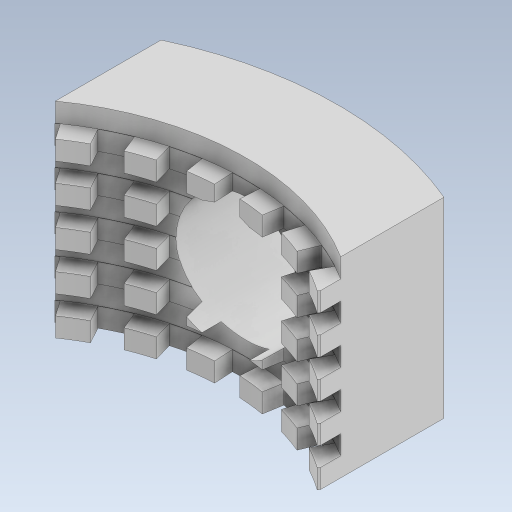
# Autodesk Inventor part: Plunger Cap
Saved by Autodesk Inventor 2023 (Build 270158000, 158)
## iProperties
Created: 2022-09-14
Part Number: Plunger Cap
Material: Generic
Document SubType Name: Modeling
Designer: Dave
Density: 1 g/cm^3
Appearance: Default
Author: Dave
Autodesk Inventor part; units mm, degrees
ref_plane "YZ Plane" through (0, 0, 0) normal (1, 0, 0) x (0, 1, 0)
ref_plane "XZ Plane" through (0, 0, 0) normal (0, 1, 0) x (-1, 0, 0)
ref_plane "XY Plane" through (0, 0, 0) normal (0, 0, 1) x (1, 0, 0)
sketch "Sketch1" plane through (0, 0, 0) normal (0, 1, 0) x (-1, 0, 0)
  arc A0 (16.223, 7.3) -> (7.325, 16.198) centre (0, -0.025) ccw
  line L0 (7.325, 16.198) -> (7.325, 21.125)
  arc A1 (7.325, 21.125) -> (7.025, 22.1786) centre (5.325, 21.125) ccw
  arc A2 (7.025, 22.1786) -> (6.3786, 22.825) centre (5.325, 21.125) ccw
  arc A3 (6.3786, 22.825) -> (5.325, 23.125) centre (5.325, 21.125) ccw
  line L1 (5.325, 23.125) -> (-5.325, 23.125)
  arc A4 (-5.325, 23.125) -> (-6.3786, 22.825) centre (-5.325, 21.125) ccw
  arc A5 (-6.3786, 22.825) -> (-7.025, 22.1786) centre (-5.325, 21.125) ccw
  arc A6 (-7.025, 22.1786) -> (-7.325, 21.125) centre (-5.325, 21.125) ccw
  line L2 (-7.325, 21.125) -> (-7.325, 16.198)
  arc A7 (-7.325, 16.198) -> (-16.223, 7.3) centre (0, -0.025) ccw
  line L3 (-16.223, 7.3) -> (-21.1473, 7.3)
  ellipse E0 centre (-21.2521, 5.3) end of major axis (-19.7618, 6.7142) minor radius 1.9496 (-21.1473, 7.3) -> (-22.218, 7) ccw
  ellipse E1 centre (-21.163, 5.3) end of major axis (-23.1657, 5.3) minor radius 2 (-22.218, 7) -> (-22.85, 6.3778) ccw
  ellipse E2 centre (-21.247, 5.3) end of major axis (-21.247, 7.3) minor radius 1.903 (-22.85, 6.3778) -> (-23.15, 5.3) ccw
  line L4 (-23.15, 5.3) -> (-23.15, -5.35)
  ellipse E3 centre (-21.247, -5.35) end of major axis (-21.247, -3.35) minor radius 1.903 (-23.15, -5.35) -> (-22.85, -6.4278) ccw
  ellipse E4 centre (-21.163, -5.35) end of major axis (-23.1657, -5.35) minor radius 2 (-22.85, -6.4278) -> (-22.218, -7.05) ccw
  ellipse E5 centre (-21.2521, -5.35) end of major axis (-22.7423, -3.9358) minor radius 1.9496 (-22.218, -7.05) -> (-21.1473, -7.35) ccw
  line L5 (-21.1473, -7.35) -> (-16.223, -7.35)
  arc A8 (-16.223, -7.35) -> (-7.325, -16.248) centre (0, -0.025) ccw
  line L6 (-7.325, -16.248) -> (-7.325, -21.175)
  line L7 (-7.025, -22.2286) -> (-7.025, -16.0531)
  arc A9 (-7.325, -21.175) -> (-7.025, -22.2286) centre (-5.325, -21.175) ccw
  arc A10 (-7.025, -22.2286) -> (-6.3786, -22.875) centre (-5.325, -21.175) ccw
  arc A11 (-6.3786, -22.875) -> (-5.325, -23.175) centre (-5.325, -21.175) ccw
  line L8 (-5.325, -23.175) -> (5.325, -23.175)
  line L9 (7.325, -21.175) -> (7.325, -16.248)
  arc A12 (7.025, -22.2286) -> (7.325, -21.175) centre (5.325, -21.175) ccw
  arc A13 (6.3786, -22.875) -> (7.025, -22.2286) centre (5.325, -21.175) ccw
  arc A14 (5.325, -23.175) -> (6.3786, -22.875) centre (5.325, -21.175) ccw
  arc A15 (7.325, -16.248) -> (16.223, -7.35) centre (0, -0.025) ccw
  line L10 (16.223, -7.35) -> (21.1473, -7.35)
  ellipse E6 centre (21.2521, -5.35) end of major axis (19.7618, -6.7642) minor radius 1.9496 (21.1473, -7.35) -> (22.218, -7.05) ccw
  ellipse E7 centre (21.163, -5.35) end of major axis (23.1657, -5.35) minor radius 2 (22.218, -7.05) -> (22.85, -6.4278) ccw
  ellipse E8 centre (21.247, -5.35) end of major axis (21.247, -7.35) minor radius 1.903 (22.85, -6.4278) -> (23.15, -5.35) ccw
  line L11 (23.15, -5.35) -> (23.15, 5.3)
  ellipse E9 centre (21.247, 5.3) end of major axis (21.247, 3.3) minor radius 1.903 (23.15, 5.3) -> (22.85, 6.3778) ccw
  ellipse E10 centre (21.163, 5.3) end of major axis (23.1657, 5.3) minor radius 2 (22.85, 6.3778) -> (22.218, 7) ccw
  ellipse E11 centre (21.2521, 5.3) end of major axis (22.7423, 3.8858) minor radius 1.9496 (22.218, 7) -> (21.1473, 7.3) ccw
  line L12 (21.1473, 7.3) -> (16.223, 7.3)
  circle A16 centre (0, -0.025) radius 13
  point P0 (0, 0)
  point P1 (0, 0)
  dimension "d0" = 26
  constraints: 32 point on circle, 26 end point, 17 centre point, 1 coincident, 1 vertical, 49 other
  measures "d0" diameter of A16
extrude "Extrusion1" add sketch "Sketch1" along normal blind 6
sketch "Sketch2" plane through (0, 6, 0) normal (0, 1, 0) x (1, 0, 0)
  circle A0 centre (0, 0.025) radius 13 projected
  line L0 (-13, 0.025) -> (-17.8, 0.025)
  arc A1 (17.8, 0.025) -> (-17.8, 0.025) centre (0, 0.025) ccw
  arc A2 (-7.325, 16.248) -> (-16.223, 7.35) centre (0, 0.025) ccw projected
  line L1 (13, 0.025) -> (17.8, 0.025)
  line L2 (-15.4153, 8.925) -> (-10.3923, 6.025)
  line L3 (10.3923, 6.025) -> (15.4153, 8.925)
  arc A3 (16.223, 7.35) -> (7.325, 16.248) centre (0, 0.025) ccw projected
  line L4 (0, 32.435) -> (0, -32.385) projected
  circle A4 centre (0, 0.025) radius 12
  point P0 (0, 0)
  point P1 (-11.2583, 6.525)
  point P2 (11.2583, 6.525)
  dimension "d3" = 120
  dimension "d6" = 1
  constraints: 10 point on circle, 8 end point, 2 centre point, 2 coincident, 2 horizontal, 2 horizontal alignment, 2 point on line, 1 concentric, 1 line through centre, 1 other
  measures "d3" angle of L3 L2
  measures "d6" radial gap between concentric circles of A0 A4
extrude "Extrusion2" add sketch "Sketch2" along normal blind 10 contours L3 A4 L4 A0 | A0 L4 A1 L3 | L4 A4 L2 A0 | A0 L2 A1 L4 picked at (10.4372, 7.0912) picked at (-10.4372, 7.0912)
sketch "Sketch3" plane through (0, 16, 0) normal (0, 1, 0) x (1, 0, 0)
  arc A0 (10.3923, 6.025) -> (-10.3923, 6.025) centre (0, 0.025) ccw projected
  circle A1 centre (0, 0) radius 12.0125
  line L0 (-11.2583, 6.525) -> (-10.3923, 6.025) projected
  circle A2 centre (0, 0) radius 13.0125
  line L1 (-10.3923, 6.025) -> (-11.2583, 6.525)
  arc A3 (11.2583, 6.525) -> (-11.2583, 6.525) centre (0, 0.025) ccw projected
  line L2 (-9.6664, 7.1317) -> (-10.4722, 7.7239)
  line L3 (-8.8232, 8.1518) -> (-9.5589, 8.8291)
  line L4 (-7.8729, 9.0729) -> (-8.5297, 9.827)
  line L5 (-6.827, 9.8839) -> (-7.3968, 10.7057)
  line L6 (-5.6983, 10.575) -> (-6.1742, 11.4545)
  line L7 (-4.5004, 11.1377) -> (-4.8767, 12.0642)
  line L8 (-3.2478, 11.5651) -> (-3.5199, 12.5274)
  line L9 (-1.9558, 11.8522) -> (-2.1204, 12.8386)
  line L10 (-0.6401, 11.9955) -> (-0.6952, 12.9939)
  line L11 (0.6834, 11.9931) -> (0.7384, 12.9915)
  line L12 (1.9985, 11.8451) -> (2.1631, 12.8315)
  line L13 (3.2895, 11.5534) -> (3.5616, 12.5156)
  line L14 (4.5405, 11.1214) -> (4.9168, 12.0479)
  line L15 (5.7364, 10.5544) -> (6.2123, 11.4338)
  line L16 (6.8626, 9.8593) -> (7.4324, 10.681)
  line L17 (7.9056, 9.0445) -> (8.5623, 9.7986)
  line L18 (8.8525, 8.1199) -> (9.5883, 8.7972)
  line L19 (9.6921, 7.0968) -> (10.4978, 7.689)
  line L20 (10.414, 5.9875) -> (11.28, 6.4875)
  point P0 (0.0028, 0.0248)
  point P1 (0.0055, 0.0244)
  point P2 (0.0081, 0.0236)
  point P3 (0.0107, 0.0226)
  point P4 (0.0131, 0.0213)
  point P5 (0.0154, 0.0197)
  point P6 (0.0174, 0.0179)
  point P7 (0.0193, 0.0159)
  point P8 (0.0209, 0.0137)
  point P9 (0.0223, 0.0113)
  point P10 (0.0234, 0.0088)
  point P11 (0.0242, 0.0061)
  point P12 (0.0248, 0.0034)
  point P13 (0.025, 0.0007)
  point P14 (0.0249, -0.0021)
  point P15 (0.0245, -0.0048)
  point P16 (0.0239, -0.0075)
  point P17 (0.0229, -0.01)
  point P18 (0.0217, -0.0125)
  point P19 (9.6939, 7.0981)
  point P20 (8.8558, 8.1229)
  point P21 (7.9097, 9.0492)
  point P22 (6.8672, 9.8658)
  point P23 (5.7409, 10.5627)
  point P24 (4.5445, 11.1312)
  point P25 (3.2926, 11.5644)
  point P26 (2.0005, 11.8571)
  point P27 (0.684, 12.0055)
  point P28 (-0.6408, 12.0079)
  point P29 (-1.9578, 11.8642)
  point P30 (-3.251, 11.5762)
  point P31 (-4.5044, 11.1475)
  point P32 (-5.7028, 10.5833)
  point P33 (-6.8316, 9.8906)
  point P34 (-7.8771, 9.0777)
  point P35 (-8.8265, 8.1548)
  point P36 (-9.6683, 7.133)
  dimension "d9" = 120
  constraints: 40 end point, 3 point on circle, 2 coincident, 1 centre point, 80 other
extrude "Extrusion3" cut sketch "Sketch3" against normal blind 10 contours A0 L18 A2 L19 | A0 L16 A2 L17 | L2 A2 L3 A0 | A0 L14 A2 L15 | L4 A2 L5 A0 | A0 L12 A2 L13 | L6 A2 L7 A0 | A0 L10 A2 L11 | L8 A2 L9 A0
sketch "Sketch4" plane through (15.4153, 6, -8.925) normal (0.5, 0, 0.8660254) x (0.8660254, 0, -0.5)
  line L0 (-5.8, 10) -> (0, 10) projected
  line L1 (-5.8, 10) -> (-4.8, 10)
  line L2 (-5.8, 0) -> (-4.8, 0) projected
  line L3 (-5.8, 10) -> (-5.8, 0)
  line L4 (-5.8, 0) -> (-4.8, 0)
  line L5 (-5.498, 10) -> (-5.498, 0) projected
  line L6 (-4.8, 0) -> (-4.8, 10)
  line L7 (-5.8, 9) -> (-4.8, 9)
  line L8 (-5.8, 8) -> (-4.8, 8)
  line L9 (-5.8, 7) -> (-4.8, 7)
  line L10 (-5.8, 6) -> (-4.8, 6)
  line L11 (-5.8, 5) -> (-4.8, 5)
  line L12 (-5.8, 4) -> (-4.8, 4)
  line L13 (-5.8, 3) -> (-4.8, 3)
  line L14 (-5.8, 2) -> (-4.8, 2)
  line L15 (-5.8, 1) -> (-4.8, 1)
  line L16 (-17.8125, -9.2) -> (-17.8125, 13.2) projected
  line L17 (-7.5305, 10) -> (-6.7156, 10) projected
  line L18 (-5.8, 0) -> (-6.7852, 0)
  line L19 (-6.7852, 0) -> (-6.7852, 10)
  line L20 (-6.7852, 10) -> (-5.8, 10)
  line L21 (-5.8, 10) -> (-5.8, 0)
  point P0 (-17.8125, -6)
  point P1 (-4.8, 1)
  point P2 (-4.8, 2)
  point P3 (-5.8, 2)
  point P4 (-5.8, 1)
  point P5 (-4.8, 3)
  point P6 (-4.8, 4)
  point P7 (-5.8, 4)
  point P8 (-5.8, 3)
  point P9 (-4.8, 5)
  point P10 (-4.8, 6)
  point P11 (-5.8, 6)
  point P12 (-5.8, 5)
  point P13 (-4.8, 7)
  point P14 (-4.8, 8)
  point P15 (-5.8, 8)
  point P16 (-5.8, 7)
  point P17 (-4.8, 9)
  point P18 (-4.8, 10)
  point P19 (-5.8, 9)
  dimension "d16" = 1
  constraints: 34 end point, 3 equal length, 3 vertical, 2 horizontal, 1 perpendicular, 1 point on line, 27 other
  measures "d16" distance of L0.start L7.start
revolve "Revolution1" cut sketch "Sketch4" angle 360 about axis through (-0.0108, -10, -0.0188) along (0, -1, 0) contours L0 L5 L7 L3 | L3 L18 L19 L17 L20 | L0 L6 L7 L5 | L8 L5 L9 L3 | L8 L6 L9 L5 | L10 L5 L11 L3 | L10 L6 L11 L5 | L3 L14 L5 L15 | L12 L5 L13 L3 | L5 L14 L6 L15 | L12 L6 L13 L5
sketch "Sketch25" plane through (0, 0, 0) normal (0, -1, 0) x (1, 0, 0)
  line L0 (5.325, -23.175) -> (-5.325, -23.175) projected
  arc A0 (5.325, -23.175) -> (7.325, -21.175) centre (5.325, -21.175) ccw projected
  line L1 (7.325, -16.248) -> (7.325, -21.175) projected
  arc A1 (7.325, -16.248) -> (16.223, -7.35) centre (0, -0.025) ccw projected
  line L2 (21.1473, -7.35) -> (16.223, -7.35) projected
  ellipse E0 centre (21.2521, -5.35) end of major axis (22.7423, -3.9358) minor radius 1.9496 (21.1473, -7.35) -> (22.218, -7.05) ccw projected
  ellipse E1 centre (21.163, -5.35) end of major axis (23.1657, -5.35) minor radius 2 (22.218, -7.05) -> (22.85, -6.4278) ccw projected
  ellipse E2 centre (21.247, -5.35) end of major axis (21.247, -3.35) minor radius 1.903 (22.85, -6.4278) -> (23.15, -5.35) ccw projected
  line L3 (23.15, 5.3) -> (23.15, -5.35) projected
  ellipse E3 centre (21.247, 5.3) end of major axis (21.247, 7.3) minor radius 1.903 (23.15, 5.3) -> (22.85, 6.3778) ccw projected
  ellipse E4 centre (21.163, 5.3) end of major axis (23.1657, 5.3) minor radius 2 (22.85, 6.3778) -> (22.218, 7) ccw projected
  ellipse E5 centre (21.2521, 5.3) end of major axis (19.7618, 6.7142) minor radius 1.9496 (22.218, 7) -> (21.1473, 7.3) ccw projected
  line L4 (16.223, 7.3) -> (21.1473, 7.3) projected
  arc A2 (16.223, 7.3) -> (7.325, 16.198) centre (0, -0.025) ccw projected
  line L5 (7.325, 21.125) -> (7.325, 16.198) projected
  arc A3 (7.325, 21.125) -> (5.325, 23.125) centre (5.325, 21.125) ccw projected
  line L6 (-5.325, 23.125) -> (5.325, 23.125) projected
  arc A4 (-5.325, 23.125) -> (-7.325, 21.125) centre (-5.325, 21.125) ccw projected
  line L7 (-7.325, 16.198) -> (-7.325, 21.125) projected
  arc A5 (-7.325, 16.198) -> (-16.223, 7.3) centre (0, -0.025) ccw projected
  line L8 (-21.1473, 7.3) -> (-16.223, 7.3) projected
  ellipse E6 centre (-21.2521, 5.3) end of major axis (-22.7423, 3.8858) minor radius 1.9496 (-21.1473, 7.3) -> (-22.218, 7) ccw projected
  ellipse E7 centre (-21.163, 5.3) end of major axis (-23.1657, 5.3) minor radius 2 (-22.218, 7) -> (-22.85, 6.3778) ccw projected
  ellipse E8 centre (-21.247, 5.3) end of major axis (-21.247, 3.3) minor radius 1.903 (-22.85, 6.3778) -> (-23.15, 5.3) ccw projected
  line L9 (-23.15, -5.35) -> (-23.15, 5.3) projected
  ellipse E9 centre (-21.247, -5.35) end of major axis (-21.247, -7.35) minor radius 1.903 (-23.15, -5.35) -> (-22.85, -6.4278) ccw projected
  ellipse E10 centre (-21.163, -5.35) end of major axis (-23.1657, -5.35) minor radius 2 (-22.85, -6.4278) -> (-22.218, -7.05) ccw projected
  ellipse E11 centre (-21.2521, -5.35) end of major axis (-19.7618, -6.7642) minor radius 1.9496 (-22.218, -7.05) -> (-21.1473, -7.35) ccw projected
  line L10 (-16.223, -7.35) -> (-21.1473, -7.35) projected
  arc A6 (-16.223, -7.35) -> (-7.325, -16.248) centre (0, -0.025) ccw projected
  line L11 (-7.325, -21.175) -> (-7.325, -16.248) projected
  arc A7 (-7.325, -21.175) -> (-5.325, -23.175) centre (-5.325, -21.175) ccw projected
  circle A8 centre (0, -0.025) radius 13 projected
  point P0 (0, 0)
  constraints: 12 other
extrude "Extrusion13" cut sketch "Sketch25" against normal blind 6
ref_plane "Work Plane5" through (11.2583, 15.5, -6.525) normal (0.000416, 0, -0.9999999) x (0, -1, 0)
sketch "Sketch26" plane through (11.2583, 15.5, -6.525) normal (0.000416, 0, -0.9999999) x (0, -1, 0)
  line L0 (9.5, 26.6746) -> (-0.5, 26.6746) projected
  line L1 (-0.5, 0) -> (-0.5, 22.5329) projected
  circle A0 centre (4.5, 11.2664) radius 3.25
  point P0 (15.5, 11.2556)
  point P1 (-0.5, 11.2664)
  point P2 (4.5, 26.6746)
  dimension "d107" = 6.5
  constraints: 2 midpoint, 1 centre point, 1 horizontal alignment, 1 vertical alignment
  measures "d107" diameter of A0
extrude "Extrusion14" cut sketch "Sketch26" along normal through all
sketch "Sketch27" plane through (0, 16, 0) normal (0, 1, 0) x (1, 0, 0)
  line L0 (6.9393, 20.2586) -> (-7.5607, 20.2586)
  line L1 (-7.5607, 20.2586) -> (-7.5607, 0)
  line L2 (-7.5607, 0) -> (6.9393, 0)
  line L3 (6.9393, 0) -> (6.9393, 20.2586)
  line L4 (20.3406, 29.2417) -> (-23.901, 29.2417)
  line L5 (-23.901, 29.2417) -> (-23.901, -10.912)
  line L6 (-23.901, -10.912) -> (20.3406, -10.912)
  line L7 (20.3406, -10.912) -> (20.3406, 29.2417)
  point P0 (0, 0)
  point P1 (-0.3107, 0)
  dimension "d110" = 14.5
  constraints: 16 end point, 4 parallel, 2 horizontal, 2 perpendicular, 1 horizontal alignment, 1 midpoint
  measures "d110" distance of L1.end L2.end
extrude "Extrusion15" cut sketch "Sketch27" against normal through all
body "Solid1"
